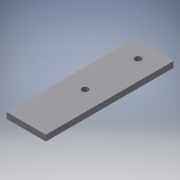
# Autodesk Inventor part: Ball screw right hand support
Saved by Autodesk Inventor 2016 (Build 200138000, 138)
## iProperties
Created: 2017-06-13
Part Number: Ball screw right hand support
Material: Generic
Document SubType Name: Modeling
Designer: m228540
Density: 1 g/cm^3
Appearance: Default
Author: m228540
Autodesk Inventor part; units mm, degrees
ref_plane "YZ Plane" through (0, 0, 0) normal (1, 0, 0) x (0, 1, 0)
ref_plane "XZ Plane" through (0, 0, 0) normal (0, 1, 0) x (-1, 0, 0)
ref_plane "XY Plane" through (0, 0, 0) normal (0, 0, 1) x (1, 0, 0)
sketch "Sketch1" plane through (0, 0, 0) normal (0, 0, 1) x (1, 0, 0)
  line L0 (-29.8485, 74.7727) -> (10.1515, 74.7727)
  line L1 (10.1515, 74.7727) -> (10.1515, -55.2273)
  line L2 (10.1515, -55.2273) -> (-29.8485, -55.2273)
  line L3 (-29.8485, -55.2273) -> (-29.8485, 74.7727)
  point P0 (0, 0)
  dimension "d0" = 40
  dimension "d1" = 130
  constraints: 8 end point, 2 parallel, 1 horizontal, 1 perpendicular
  measures "d0" distance of L1.end L2.end
  measures "d1" distance of L0.end L1.end
extrude "Extrusion1" add sketch "Sketch1" along normal blind 6
sketch "Sketch2" plane through (0, 0, 0) normal (0, 0, -1) x (-1, 0, 0)
  circle A0 centre (9.8485, 58.7727) radius 3.3 projected
  circle A1 centre (9.8485, 4.7727) radius 3.3 projected
  point P0 (0, 0)
extrude "Extrusion2" cut sketch "Sketch2" against normal through all
body "Solid1"
